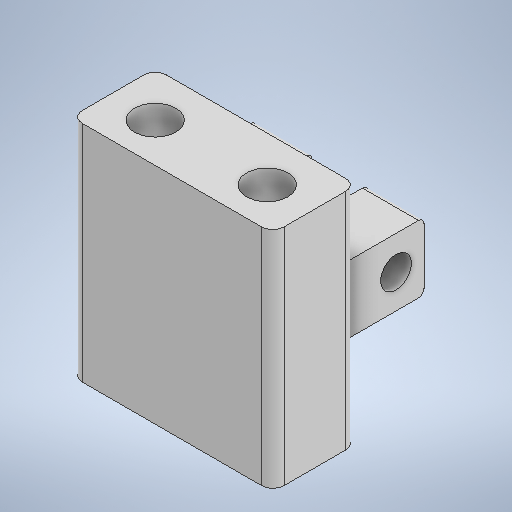
# Autodesk Inventor part: zaslepka
Saved by Autodesk Inventor 2025.2 (Build 292293000, 293)
## iProperties
Created: 2025-11-26
Part Number: zaslepka
Material: Ogólny
Document SubType Name: Modeling
Designer: juras
Density: 1 g/cm^3
Appearance: Domyślna
Author: juras
Autodesk Inventor part; units mm, degrees
ref_plane "YZ Plane" through (0, 0, 0) normal (1, 0, 0) x (0, 1, 0)
ref_plane "XZ Plane" through (0, 0, 0) normal (0, 1, 0) x (-1, 0, 0)
ref_plane "XY Plane" through (0, 0, 0) normal (0, 0, 1) x (1, 0, 0)
sketch "Szkic2" plane through (0, 0, 0) normal (0, 1, 0) x (-1, 0, 0)
  line L0 (-20, -7.5) -> (20, -7.5)
  line L1 (20, -7.5) -> (20, 7.5)
  line L2 (20, 7.5) -> (-20, 7.5)
  line L3 (-20, 7.5) -> (-20, -7.5)
  line L4 (-20, -7.5) -> (20, 7.5) construction
  line L5 (20, -7.5) -> (-20, 7.5) construction
  point P0 (0, 0)
  dimension "d12" = 40
  dimension "d13" = 15
  constraints: 12 end point, 2 midpoint, 2 parallel, 1 horizontal, 1 perpendicular
  measures "d12" distance of L2.end L1.end
  measures "d13" distance of L1.end L0.end
extrude "Wyciągnięcie proste1" add sketch "Szkic2" along normal mid plane 20
sketch "Szkic3" plane through (0, 10, 0) normal (0, 1, 0) x (1, 0, 0)
  line L0 (18, 7.5) -> (-18, 7.5)
  line L1 (-18, 7.5) -> (-18, -7.5)
  line L2 (-18, -7.5) -> (18, -7.5)
  line L3 (18, -7.5) -> (18, 7.5)
  line L4 (18, 7.5) -> (-18, -7.5) construction
  line L5 (-18, 7.5) -> (18, -7.5) construction
  circle A0 centre (10, -0.5) radius 6
  circle A1 centre (-10, -0.5) radius 6
  circle A2 centre (10, -0.5) radius 3.7
  circle A3 centre (-10, -0.5) radius 3.7
  line L6 (-20, -7.5) -> (20, -7.5) projected
  point P0 (0, 0)
  point P1 (10, -7)
  point P2 (10, 8)
  point P3 (-13.3166, 8)
  point P4 (-10, -7)
  point P5 (15.1962, -4)
  point P6 (-15.1962, -4)
  dimension "d16" = 36
  dimension "d17" = 15
  dimension "d18" = 12
  dimension "d19" = 8
  dimension "d20" = 8
  dimension "d21" = 12
  dimension "d22" = 8
  dimension "d23" = 8
  dimension "d24" = 7.4
  dimension "d25" = 7.4
  constraints: 12 end point, 4 centre point, 2 coincident, 2 midpoint, 2 parallel, 1 horizontal, 1 perpendicular
  measures "d16" distance of L2.end L1.end
  measures "d17" distance of L1.end L0.end
  measures "d18" diameter of A0
  measures "d19" distance from line of A0.centre L3
  measures "d20" distance from line of L0 A0.centre
  measures "d21" diameter of A1
  measures "d22" distance from line of L0 A1.centre
  measures "d23" distance from line of L1 A1.centre
  measures "d24" diameter of A2
  measures "d25" diameter of A3
fillet "Zaokrąglenie1" radius 2 4 edges at (20, 0, 7.5) (-20, 0, 7.5) (20, 0, -7.5) (-20, 0, -7.5)
extrude "Wyciągnięcie proste3" add sketch "Szkic3" along normal blind 20 contours L3 L2 L1 L0 | A0 | A1
sketch "Szkic4" plane through (18, 10, -7.5) normal (0, 0, -1) x (-1, 0, 0)
  line L0 (33, 0) -> (23, -20) construction
  line L1 (23, 0) -> (33, -20) construction
  line L2 (13, 6) -> (3, 6)
  line L3 (3, 6) -> (3, -6)
  line L4 (3, -6) -> (13, -6)
  line L5 (13, -6) -> (13, 6)
  line L6 (13, 6) -> (3, -6) construction
  line L7 (3, 6) -> (13, -6) construction
  line L8 (36, -20) -> (0, -20) projected
  line L9 (0, 0) -> (36, 0) projected
  line L10 (-2, 0) -> (-2, -20) projected
  line L11 (0, 20) -> (36, 20) projected
  point P0 (18, -10)
  point P1 (28, -10)
  point P2 (8, 0)
  dimension "d32" = 14
  dimension "d38" = 10
  dimension "d39" = 5
  dimension "d68" = 14
  constraints: 16 end point, 4 midpoint, 2 parallel, 1 horizontal, 1 perpendicular
  measures "d32" distance between parallel lines of L8 L4
  measures "d38" distance between parallel lines of L5 L3
  measures "d39" distance between parallel lines of L10 L3
  measures "d68" distance between parallel lines of L2 L11
extrude "Wyciągnięcie proste4" add sketch "Szkic4" along normal blind 15
sketch "Szkic7" plane through (5, 4, -7.5) normal (-1, 0, 0) x (0, 0, 1)
  line L0 (-15, 12) -> (-15, 0) projected
  line L1 (-15, 0) -> (-15, 3)
  line L2 (0, -14) -> (0, 6) projected
  line L3 (0, 0) -> (-15, 0) projected
  line L4 (0, 0) -> (-15, 0)
  line L5 (-15, 12) -> (-15, 9)
  line L6 (0, 12) -> (-15, 12) projected
  line L7 (0, 12) -> (-15, 12)
  circle A0 centre (-10, 6) radius 2.75
  point P0 (7.5, -4)
  dimension "d48" = 5.5
  dimension "d49" = 6
  dimension "d69" = 5
  constraints: 8 end point, 4 point on line, 2 collinear, 1 centre point
  measures "d48" diameter of A0
  measures "d49" distance from line of A0.centre L3
  measures "d69" distance from line of L0 A0.centre
extrude "Wyciągnięcie proste6" cut sketch "Szkic7" against normal blind 15
mirror "Odbij1" about plane through (0, 0, 0) normal (1, 0, 0) of "Wyciągnięcie proste6", "Wyciągnięcie proste4"
sketch "Szkic11" plane through (0, 10, 0) normal (0, 1, 0) x (1, 0, 0)
  line L0 (18, -7.5) -> (-18, -7.5) projected
  line L1 (18, -7.5) -> (20, -7.5)
  line L2 (20, -7.5) -> (20, 7.5)
  line L3 (20, 7.5) -> (18, 7.5)
  line L4 (18, 7.5) -> (18, -7.5)
  point P0 (0, 0)
  dimension "d63" = 2
  dimension "d64" = 15
  constraints: 8 end point, 2 parallel, 1 horizontal, 1 perpendicular
  measures "d63" distance of L3.end L2.end
  measures "d64" distance of L2.end L1.end
extrude "Wyciągnięcie proste7" cut sketch "Szkic11" against normal blind 20
mirror "Odbij3" about plane through (0, 0, 0) normal (1, 0, 0) of "Wyciągnięcie proste7"
fillet "Zaokrąglenie4" radius 2 4 edges at (-18, 10, 7.5) (-18, 10, -7.5) (18, 10, -7.5) (18, 10, 7.5)
fillet "Zaokrąglenie5" radius 1 4 edges at (-10, 16, -22.5) (-10, 4, -22.5) (10, 4, -22.5) (10, 16, -22.5)
fillet "Zaokrąglenie6" radius 1 8 edges at (-15, 10, -7.5) (-10, 16, -7.5) (-10, 4, -7.5) (-5, 10, -7.5) (10, 4, -7.5) (5, 10, -7.5) (15, 10, -7.5) (10, 16, -7.5)
sketch "Szkic12" plane through (10, 10, 0.5) normal (0, 1, 0) x (1, 0, 0)
  circle A0 centre (0, 0) radius 3.7
  point P0 (-10, 0.5)
  constraints: 1 centre point
extrude "Wyciągnięcie proste8" cut sketch "Szkic12" against normal blind 44
mirror "Odbij4" about plane through (0, 0, 0) normal (1, 0, 0) of "Wyciągnięcie proste8"
